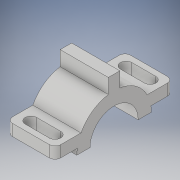
# Autodesk Inventor part: 練習一
Saved by Autodesk Inventor 2017 (Build 210142000, 142)
## iProperties
Part Number: 練習一
Material: 一般
Document SubType Name: Modeling
Designer: user
Density: 1 g/cm^3
Appearance: 預設
Author: user
Autodesk Inventor part; units mm, degrees
ref_plane "YZ Plane" through (0, 0, 0) normal (1, 0, 0) x (0, 1, 0)
ref_plane "XZ Plane" through (0, 0, 0) normal (0, 1, 0) x (-1, 0, 0)
ref_plane "XY Plane" through (0, 0, 0) normal (0, 0, 1) x (1, 0, 0)
sketch "草圖1" plane through (0, 0, 0) normal (1, 0, 0) x (0, 1, 0)
  arc A0 (0, -21) -> (0, 21) centre (0, 0) ccw
  line L0 (0, 33.7624) -> (0, -28.793) construction
  line L1 (0, -21) -> (0, -32.5)
  line L2 (15, -28.8314) -> (15, -51.5)
  line L3 (5, -51.5) -> (5, -32.1131)
  arc A1 (0, -32.5) -> (5, -32.1131) centre (0, 0) ccw
  line L4 (5, -51.5) -> (15, -51.5)
  line L5 (0, 0) -> (31.6672, 0)
  line L6 (45, -5) -> (32.1131, -5)
  line L7 (45, -5) -> (45, 0)
  arc A2 (15, -28.8314) -> (32.1131, -5) centre (0, 0) ccw
  line L8 (45, 5) -> (32.1131, 5)
  line L9 (45, 5) -> (45, 0)
  line L10 (15, 28.8314) -> (15, 51.5)
  line L11 (5, 51.5) -> (5, 32.1131)
  line L12 (5, 51.5) -> (15, 51.5)
  arc A3 (32.1131, 5) -> (15, 28.8314) centre (0, 0) ccw
  arc A4 (5, 32.1131) -> (0, 32.5) centre (0, 0) ccw
  line L13 (0, 32.5) -> (0, 21)
  dimension "d0" = 10
  dimension "d2" = 45
  dimension "d4" = 10
  dimension "d6" = 42
  dimension "d7" = 65
  dimension "d9" = 103
  dimension "d10" = 5
  constraints: 28 end point, 10 point on circle, 6 point on line, 6 symmetric about line, 5 centre point, 3 horizontal, 3 vertical, 2 coincident, 1 collinear, 1 concentric, 1 perpendicular
  measures "d0" distance of L6.start L8.start
  measures "d2" distance between parallel lines of L7 L0
  measures "d4" distance of L3.start L2.end
  measures "d6" distance of L1.start L13.end
  measures "d7" distance of L1.end L13.start
  measures "d9" distance between parallel lines of L4 L12
  measures "d10" distance from line of L3 L0.end
extrude "擠出1" add sketch "草圖1" along normal blind 42
fillet "圓角1" radius 5 4 edges at (42, 10, 51.5) (0, 10, 51.5) (42, 10, -51.5) (0, 10, -51.5)
sketch "草圖2" plane through (0, 15, 28.8314) normal (0, 1, 0) x (1, 0, 0)
  arc A0 (11, -7.6686) -> (11, -17.6686) centre (11, -12.6686) ccw
  arc A1 (32, -17.6686) -> (32, -7.6686) centre (32, -12.6686) ccw
  line L0 (32, -7.6686) -> (11, -7.6686)
  line L1 (11, -17.6686) -> (32, -17.6686)
  line L2 (42, 0) -> (42, -17.6686) projected
  line L3 (0, 28.8314) -> (45.6948, 28.8314)
  arc A2 (11, 75.3314) -> (11, 65.3314) centre (11, 70.3314) ccw
  arc A3 (32, 65.3314) -> (32, 75.3314) centre (32, 70.3314) ccw
  line L4 (32, 65.3314) -> (11, 65.3314)
  line L5 (11, 75.3314) -> (32, 75.3314)
  line L6 (5, -22.6686) -> (37, -22.6686) projected
  point P0 (42, 75.3314)
  dimension "d14" = 10
  dimension "d15" = 21
  dimension "d16" = 10
  dimension "d17" = 83
  constraints: 10 end point, 8 point on circle, 7 symmetric about line, 4 centre point, 3 horizontal, 3 tangent, 1 equal radius, 2 other
  measures "d14" distance between parallel lines of L0 L1
  measures "d15" distance of A1.centre A0.centre
  measures "d16" distance from line of L2 A1.centre
  measures "d17" distance of A2.centre A0.centre
extrude "擠出2" cut sketch "草圖2" against normal blind 42
